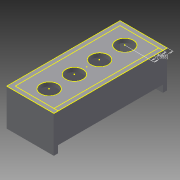
# Autodesk Inventor part: SwitchPanel
Saved by Autodesk Inventor 2015 (Build 190159000, 159)
## iProperties
Created: 2015-04-05
Part Number: SwitchPanel
Material: Generic
Document SubType Name: Modeling
Designer: Judson
Density: 1 g/cm^3
Appearance: Default
Author: Judson
Autodesk Inventor part; units mm, degrees
ref_plane "YZ Plane" through (0, 0, 0) normal (1, 0, 0) x (0, 1, 0)
ref_plane "XZ Plane" through (0, 0, 0) normal (0, 1, 0) x (-1, 0, 0)
ref_plane "XY Plane" through (0, 0, 0) normal (0, 0, 1) x (1, 0, 0)
sketch "Sketch1" plane through (0, 0, 0) normal (0, 1, 0) x (-1, 0, 0)
  line L0 (39.995, 16.6749) -> (-40.005, 16.6749)
  line L1 (-40.005, 16.6749) -> (-40.005, -16.6751)
  line L2 (-40.005, -16.6751) -> (39.995, -16.6751)
  line L3 (39.995, -16.6751) -> (39.995, 16.6749)
  circle A0 centre (-26.67, -0.0001) radius 6.1
  circle A1 centre (-8.89, -0.0001) radius 6.1
  circle A2 centre (8.89, -0.0001) radius 6.1
  circle A3 centre (26.67, -0.0001) radius 6.1
  point P0 (0, 0)
  dimension "d0" = 33.35
  dimension "d1" = 80
  dimension "d2" = 16.6751
  dimension "d3" = 40.005
  dimension "d4" = 12.2
  dimension "d5" = 13.335
  dimension "d8" = 17.78
  constraints: 8 end point, 4 centre point, 2 horizontal, 2 parallel, 1 perpendicular, 6 other
  measures "d0" distance of L0.end L1.end
  measures "d1" distance of L1.end L2.end
  measures "d2" distance from line of L2 point (0, 0)
  measures "d3" distance from line of L1 point (0, 0)
  measures "d4" diameter of A0
  measures "d5" distance from line of A0.centre L1
  measures "d8" distance of A0.centre A1.centre
extrude "Extrusion1" add sketch "Sketch1" along normal blind 3
sketch "Sketch2" plane through (0, 0, 0) normal (0, -1, 0) x (1, 0, 0)
  circle A0 centre (-26.67, -0.0001) radius 6.1 projected
  circle A1 centre (-8.89, -0.0001) radius 6.1 projected
  circle A2 centre (8.89, -0.0001) radius 6.1 projected
  circle A3 centre (26.67, -0.0001) radius 6.1 projected
  line L0 (-39.995, -16.6751) -> (-39.995, 16.6749) projected
  line L1 (-39.995, 16.6749) -> (40.005, 16.6749) projected
  line L2 (40.005, 16.6749) -> (40.005, -16.6751) projected
  line L3 (40.005, -16.6751) -> (-39.995, -16.6751) projected
  line L4 (36.995, -13.6749) -> (-36.995, -13.6749)
  line L5 (-36.995, -13.6749) -> (-36.995, 13.6749)
  line L6 (-36.995, 13.6749) -> (36.995, 13.6749)
  line L7 (36.995, 13.6749) -> (36.995, -13.6749)
  line L8 (36.995, -13.6749) -> (-36.995, 13.6749) construction
  line L9 (-36.995, -13.6749) -> (36.995, 13.6749) construction
  point P0 (0, 0)
  dimension "d15" = 3
  dimension "d16" = 3.01
  dimension "d17" = 3
  dimension "d18" = 10.325
  constraints: 12 end point, 2 midpoint, 2 parallel, 1 horizontal, 1 perpendicular
  measures "d15" distance between parallel lines of L0 L5
  measures "d16" distance between parallel lines of L2 L7
  measures "d17" distance between parallel lines of L1 L6
  measures "d18" distance from line of L7 A3.centre
extrude "Extrusion2" add sketch "Sketch2" along normal blind 23 contours L0 L1 L2 L3
sketch "Sketch4" plane through (-39.995, 3, 16.6749) normal (0, 0, 1) x (1, 0, 0)
  line L0 (80, -26) -> (0, -26) projected
  line L1 (0, -26) -> (0, 0) projected
  line L2 (0, 0) -> (80, 0) projected
  line L3 (80, 0) -> (80, -26) projected
  line L4 (0, 0) -> (80, 0) projected
  line L5 (3, 0) -> (3, -26)
  line L6 (76.99, 0) -> (76.99, -26)
  line L7 (76.99, -3) -> (76.99, -26) projected
  line L8 (3, -21) -> (76.99, -21)
  point P0 (39.995, -3)
  dimension "d21" = 3
  dimension "d22" = 3.01
  dimension "d23" = 5
  constraints: 6 end point, 5 point on line, 1 collinear, 1 horizontal, 1 perpendicular
  measures "d21" distance between parallel lines of L1 L5
  measures "d22" distance between parallel lines of L3 L6
  measures "d23" distance between parallel lines of L0 L8
extrude "Extrusion3" cut sketch "Sketch4" against normal blind 23 contours L0 L5 L8 L6
sketch "Sketch5" plane through (0, 3, 0) normal (0, 1, 0) x (1, 0, 0)
  circle A0 centre (-26.67, 0.0001) radius 6.1 projected
  circle A1 centre (-8.89, 0.0001) radius 6.1 projected
  circle A2 centre (8.89, 0.0001) radius 6.1 projected
  circle A3 centre (26.67, 0.0001) radius 6.1 projected
  line L0 (-39.995, -16.6749) -> (-39.995, 16.6751) projected
  line L1 (-39.995, 16.6751) -> (40.005, 16.6751) projected
  line L2 (40.005, 16.6751) -> (40.005, -16.6749) projected
  line L3 (40.005, -16.6749) -> (-39.995, -16.6749) projected
  line L4 (-36.995, 13.6749) -> (-36.995, -16.6749) projected
  line L5 (36.995, -13.6749) -> (-36.995, -13.6749) projected
  line L6 (36.995, 13.6749) -> (-36.995, 13.6749) projected
  line L7 (36.995, -16.6749) -> (36.995, 13.6749) projected
  point P0 (0, 0)
  dimension "d26" = 13.335
  dimension "d27" = 10.325
  measures "d26" distance from line of L2 A3.centre
  measures "d27" distance from line of L7 A3.centre
body "Solid1"
